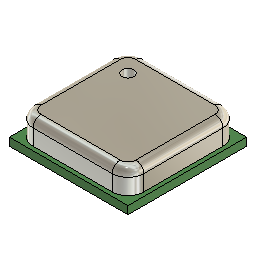
ENS160 Mox Gas (Autodesk Fusion 360 design; units mm, degrees)
Autodesk Fusion 360 part; units mm, degrees
sketch "Sketch1" plane through (0, 0, 0) normal (0, 0, 1) x (1, 0, 0)
  line L0 (-1.5, 1.5) -> (1.5, 1.5)
  line L1 (1.5, 1.5) -> (1.5, -1.5)
  line L2 (1.5, -1.5) -> (-1.5, -1.5)
  line L3 (-1.5, -1.5) -> (-1.5, 1.5)
  line L4 (0, 1.5) -> (0, 0) construction
  line L5 (0, 0) -> (-1.5, 0) construction
  dimension "d1" = 3
  constraint horizontal L0
  constraint vertical L1
  constraint horizontal L2
  constraint vertical L3
  constraint midpoint L0 L4.start
  constraint perpendicular L0 L4
  constraint perpendicular L4 L5
  constraint midpoint L3 L5.end
  constraint coincident L4.end L5.start
  constraint equal L0 L3
  measures "d1" distance of L0.start L0.end
sketch "Sketch2" plane through (0, 0, 0) normal (0, 0, 1) x (1, 0, 0)
  line L0 (-1.4, 1.4) -> (-0.7, 1.4)
  line L1 (-0.7, 1.4) -> (-0.7, 0.7)
  line L2 (-0.7, 0.7) -> (-1.4, 0.7)
  line L3 (-1.4, 0.7) -> (-1.4, 1.4)
  line L4 (-1.05, 1.4) -> (-1.05, 1.05) construction
  line L5 (-1.05, 1.05) -> (-0.7, 1.05) construction
  line L6 (0.35, 0.7) -> (-0.35, 0.7)
  line L7 (-0.35, 0.7) -> (-0.35, 1.4)
  line L8 (-0.35, 1.4) -> (0.35, 1.4)
  line L9 (0.35, 1.4) -> (0.35, 0.7)
  line L10 (1.4, 0.7) -> (0.7, 0.7)
  line L11 (0.7, 0.7) -> (0.7, 1.4)
  line L12 (0.7, 1.4) -> (1.4, 1.4)
  line L13 (1.4, 1.4) -> (1.4, 0.7)
  line L14 (-0.7, -0.35) -> (-1.4, -0.35)
  line L15 (-1.4, -0.35) -> (-1.4, 0.35)
  line L16 (-1.4, 0.35) -> (-0.7, 0.35)
  line L17 (-0.7, 0.35) -> (-0.7, -0.35)
  line L18 (0.35, -0.35) -> (-0.35, -0.35)
  line L19 (-0.35, -0.35) -> (-0.35, 0.35)
  line L20 (-0.35, 0.35) -> (0.35, 0.35)
  line L21 (0.35, 0.35) -> (0.35, -0.35)
  line L22 (1.4, -0.35) -> (0.7, -0.35)
  line L23 (0.7, -0.35) -> (0.7, 0.35)
  line L24 (0.7, 0.35) -> (1.4, 0.35)
  line L25 (1.4, 0.35) -> (1.4, -0.35)
  line L26 (-0.7, -1.4) -> (-1.4, -1.4)
  line L27 (-1.4, -1.4) -> (-1.4, -0.7)
  line L28 (-1.4, -0.7) -> (-0.7, -0.7)
  line L29 (-0.7, -0.7) -> (-0.7, -1.4)
  line L30 (0.35, -1.4) -> (-0.35, -1.4)
  line L31 (-0.35, -1.4) -> (-0.35, -0.7)
  line L32 (-0.35, -0.7) -> (0.35, -0.7)
  line L33 (0.35, -0.7) -> (0.35, -1.4)
  line L34 (1.4, -1.4) -> (0.7, -1.4)
  line L35 (0.7, -1.4) -> (0.7, -0.7)
  line L36 (0.7, -0.7) -> (1.4, -0.7)
  line L37 (1.4, -0.7) -> (1.4, -1.4)
  line L38 (-1.4, -1.05) -> (-1.05, -1.4)
  dimension "d3" = 0.7
  dimension "d4" = 0.7
  dimension "d5" = 1.05
  dimension "d6" = 1.05
  dimension "d9" = 1.05
  dimension "d10" = -1.05
  constraint horizontal L0
  constraint vertical L1
  constraint horizontal L2
  constraint vertical L3
  constraint midpoint L0 L4.start
  constraint perpendicular L0 L4
  constraint midpoint L1 L5.end
  constraint perpendicular L1 L5
  constraint midpoint L27 L38.start
  constraint midpoint L26 L38.end
  measures "d3" distance of L0.start L0.end
  measures "d4" distance of L0.start L2.end
  measures "d5" distance of origin L4
  measures "d6" distance of origin L5
extrude "Extrude1" add sketch "Sketch1" along normal blind 0.2 makes body 1
sketch "Sketch3" plane through (0, 0, 0.2) normal (0, 0, 1) x (-1, 0, 0)
  line L0 (1.4, -1.4) -> (-1.4, -1.4)
  line L1 (-1.4, -1.4) -> (-1.4, 1.4)
  line L2 (-1.4, 1.4) -> (1.4, 1.4)
  line L3 (1.4, 1.4) -> (1.4, -1.4)
  line L4 (0, -1.4) -> (0, 0) construction
  line L5 (0, 0) -> (1.4, 0) construction
  circle A0 centre (0.8, -0.8) radius 0.15
  dimension "d13" = 2.8
  dimension "d14" = 2.8
  dimension "d15" = 0.3
  dimension "d16" = 0.8
  dimension "d17" = 0.8
  constraint horizontal L0
  constraint vertical L1
  constraint horizontal L2
  constraint vertical L3
  constraint midpoint L0 L4.start
  constraint perpendicular L0 L4
  constraint midpoint L3 L5.end
  constraint perpendicular L3 L5
  constraint coincident L4.end L5.start
  measures "d13" distance of L0.start L0.end
  measures "d14" distance of L0.start L2.end
  measures "d15" diameter of A0
  measures "d16" distance of L4 A0.centre
  measures "d17" distance of L5 A0.centre
extrude "Extrude2" add sketch "Sketch3" along normal blind 0.6 separate body makes body 2
fillet "Fillet1" radius 0.4 4 edges at (-1.4, -1.4, 0.5) (-1.4, 1.4, 0.5) (1.4, 1.4, 0.5) (1.4, -1.4, 0.5) on bodies 2
fillet "Fillet2" radius 0.2 8 edges at (1.2828, -1.2828, 0.8) (1.4, 0, 0.8) (1.2828, 1.2828, 0.8) (0, 1.4, 0.8) (-1.2828, 1.2828, 0.8) (-1.4, 0, 0.8) (-1.2828, -1.2828, 0.8) (0, -1.4, 0.8) on bodies 2
extrude "Extrude3" cut sketch "Sketch2" along normal blind 0.1 contours L0 L1 L2 L3 | L6 L7 L8 L9 | L10 L11 L12 L13 | L14 L15 L16 L17 | L18 L19 L20 L21 | L22 L23 L24 L25 | L26 L27 L28 L29 L38 | L30 L31 L32 L33 | L34 L35 L36 L37 bodies 1
extrude "Extrude4" add sketch "Sketch2" along normal blind 0.1 separate body contours L0 L1 L2 L3 | L6 L7 L8 L9 | L10 L11 L12 L13 | L14 L15 L16 L17 | L18 L19 L20 L21 | L22 L23 L24 L25 | L26 L27 L28 L29 L38 | L30 L31 L32 L33 | L34 L35 L36 L37 makes body 3 at (1.1667, -1.1667, 0) makes body 4 at (-1.1667, 0.1167, 0) makes body 5 at (0.1167, -1.1667, 0) makes body 6 at (-0.1167, 0.1167, 0) makes body 7 at (0.9333, 0.1167, 0) makes body 8 at (-1.1667, 1.1667, 0) makes body 9 at (-1.05, -1.05, 0) makes body 10 at (0.1167, 0.9333, 0) makes body 11 at (1.1667, 0.9333, 0)
equation "d5 = ( 2.1 / 2 ) * 1 mm"
equation "d6 = ( 2.1 / 2 ) * 1 mm"
